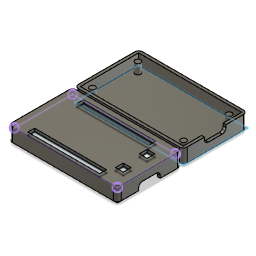
esp32-case (Autodesk Fusion 360 design; units mm, degrees)
Autodesk Fusion 360 part; units mm, degrees
sketch "Sketch1" plane through (0, 0, 0) normal (0, 1, 0) x (1, 0, 0)
  line L0 (-2, 31) -> (54, 31)
  line L1 (54, 31) -> (54, -2)
  line L2 (54, -2) -> (-2, -2)
  line L3 (-2, -2) -> (-2, 31)
  constraint horizontal L0
  constraint vertical L1
  constraint horizontal L2
  constraint vertical L3
extrude "Extrude1" add sketch "Sketch1" along normal blind 7 makes body 1
shell "Shell1" thickness 1.5 removed faces 1 at (16.6667, 7, -9) on bodies 1
cylinder "CylinderPrimitive1" add diameter 3.8 height 0.5 placed x (1, 0, 0) y (0, 0, -1) z (0, 1, 0) at (48.5, 1.5, -3.5) bodies 1
cylinder "CylinderPrimitive2" add diameter 3.8 height 3 placed x (1, 0, 0) y (0, 0, -1) z (0, 1, 0) at (48.5, 2, -3.5) bodies 1
cylinder "CylinderPrimitive3" add diameter 3 height 3 placed x (1, 0, 0) y (0, 0, -1) z (0, 1, 0) at (48.4953, 1.5, -25.4804) bodies 1
cylinder "CylinderPrimitive4" add diameter 4 height 3 placed x (1, 0, 0) y (0, 0, -1) z (0, 1, 0) at (3.5, 1.5, -25.5) bodies 1
cylinder "CylinderPrimitive5" add diameter 4 height 3 placed x (1, 0, 0) y (0, 0, -1) z (0, 1, 0) at (3.5, 1.5, -3.5) bodies 1
sketch "Sketch9" plane through (54, 0, 0) normal (1, 0, 0) x (0, 0, -1)
  line L0 (-2, 0) -> (31, 0)
  line L1 (31, 0) -> (31, 7)
  line L2 (31, 7) -> (-2, 7)
  line L3 (-2, 7) -> (-2, 0)
  line L4 (8.8903, 7) -> (8.8903, 3.7356)
  line L5 (8.8903, 3.7356) -> (20, 3.7356)
  line L6 (20, 3.7356) -> (20, 7)
  constraint coincident L2 L4.start
  constraint perpendicular L2 L4
  constraint perpendicular L4 L5
  constraint coincident L2 L6.end
  constraint perpendicular L2 L6
extrude "Extrude2" cut sketch "Sketch9" against normal blind 2 contours L2 L4 L5 L6 bodies 1
delete_face "DeleteFace1" 2 faces at (49.3668, 2.6667, -5.1908) (49.3708, 5, -2.73) on bodies 1
cylinder "CylinderPrimitive6" add diameter 4 height 3 placed x (1, 0, 0) y (0, 0, -1) z (0, 1, 0) at (48.5, 1.5, -3.5) bodies 1
delete_face "DeleteFace2" 2 faces at (48.9113, 4.5, -25.6035) (48.973, 3.5, -26.9023) on bodies 1
delete_face "DeleteFace3" 6 faces at (48.4118, 4.5, -3.9967) (50.4975, 2.5, -3.4003) (4.4276, 4.5, -2.8352) (5.4975, 2.5, -3.4003) (4.209, 4.5, -25.3143) (5.4901, 3.5, -25.3009) on bodies 1
cylinder "CylinderPrimitive7" add diameter 2.9 height 3 placed x (1, 0, 0) y (0, 0, -1) z (0, 1, 0) at (49.7786, 1.5, -2.3192) bodies 1
cylinder "CylinderPrimitive8" add diameter 2.9 height 3 placed x (1, 0, 0) y (0, 0, -1) z (0, 1, 0) at (2.2734, 1.5, -2.2495) bodies 1
cylinder "CylinderPrimitive9" add diameter 2.9 height 3 placed x (1, 0, 0) y (0, 0, -1) z (0, 1, 0) at (49.7438, 1.5, -26.8032) bodies 1
cylinder "CylinderPrimitive10" add diameter 2.9 height 3 placed x (1, 0, 0) y (0, 0, -1) z (0, 1, 0) at (2.2594, 1.5, -26.7528) bodies 1
delete_face "DeleteFace4" 4 faces at (49.9955, 2.5, -28.2312) (49.1847, 4.5, -27.2696) (50.0304, 2.5, -3.7472) (49.1826, 4.5, -2.7643) on bodies 1
delete_face "DeleteFace5" 4 faces at (3.7162, 3.5, -2.1052) (1.7425, 4.5, -2.8841) (3.7076, 2.5, -26.6805) (1.7285, 4.5, -27.3874) on bodies 1
cylinder "CylinderPrimitive11" add diameter 2.9 height 5 placed x (1, 0, 0) y (0, 0, -1) z (0, 1, 0) at (2.6, 1.5, -26) bodies 1
cylinder "CylinderPrimitive12" add diameter 2.9 height 5 placed x (1, 0, 0) y (0, 0, -1) z (0, 1, 0) at (2.6, 1.5, -2.6) bodies 1
cylinder "CylinderPrimitive13" add diameter 2.9 height 5 placed x (1, 0, 0) y (0, 0, -1) z (0, 1, 0) at (49.6109, 1.5, -2.5905) bodies 1
cylinder "CylinderPrimitive14" add diameter 2.9 height 5 placed x (1, 0, 0) y (0, 0, -1) z (0, 1, 0) at (49.6, 1.5, -26) bodies 1
fillet "Fillet1" radius 2 1 edges at (54, 3.5, -31) on bodies 1
fillet "Fillet2" radius 2 1 edges at (-2, 3.5, -31) on bodies 1
fillet "Fillet3" radius 2 1 edges at (-2, 3.5, 2) on bodies 1
fillet "Fillet4" radius 2 1 edges at (54, 3.5, 2) on bodies 1
fillet "Fillet5" radius 2 1 edges at (53.25, 3.7356, -8.8903) on bodies 1
fillet "Fillet6" radius 2 1 edges at (53.25, 3.7356, -20) on bodies 1
copy_body "CopyPasteBodies1" bodies 1 makes body 2
move_body "Move1" bodies 2 to x (1, 0, 0) y (0, -1, 0) z (0, 0, -1) at (0, 7, 5)
copy_body "Body->Comp1" bodies 2 removing the originals makes body 3 in component "Lid"
sketch "Sketch28" plane through (0, 5.5, 0) normal (0, -1, 0) x (1, 0, 0)
  circle A0 centre (49.6, 31) radius 1.45
  circle A1 centre (49.6109, 7.5905) radius 1.45
  circle A2 centre (2.6, 7.6) radius 1.45
  circle A3 centre (2.6, 31) radius 1.45
  line L0 (-0.5, 4.5) -> (52.5, 4.5)
  line L1 (52.5, 4.5) -> (52.5, 34.5)
  line L2 (52.5, 34.5) -> (-0.5, 34.5)
  line L3 (-0.5, 34.5) -> (-0.5, 4.5)
  line L4 (-0.5, 34.5) -> (2.6, 34.5)
  line L5 (2.6, 34.5) -> (2.6, 31)
  line L6 (2.6, 31) -> (-0.5, 31)
  line L7 (-0.5, 31) -> (-0.5, 34.5)
  circle A4 centre (2.6, 31) radius 1.45
  line L8 (2.6, 7.6) -> (-0.5, 7.6)
  line L9 (-0.5, 7.6) -> (-0.5, 4.5)
  line L10 (-0.5, 4.5) -> (2.6, 4.5)
  line L11 (2.6, 4.5) -> (2.6, 7.6)
  line L12 (49.6, 31) -> (52.5, 31)
  line L13 (52.5, 31) -> (52.5, 34.5)
  line L14 (52.5, 34.5) -> (49.6, 34.5)
  line L15 (49.6, 34.5) -> (49.6, 31)
  line L16 (49.6109, 7.5905) -> (52.5, 7.5905)
  line L17 (52.5, 7.5905) -> (52.5, 4.5)
  line L18 (52.5, 4.5) -> (49.6109, 4.5)
  line L19 (49.6109, 4.5) -> (49.6109, 7.5905)
  dimension "d47" = 3.1
  dimension "d48" = 3.5
  constraint horizontal L4
  constraint vertical L5
  constraint horizontal L6
  constraint vertical L7
  constraint coincident L2.end L3.start
  constraint concentric A3 A4
  constraint horizontal L8
  constraint vertical L9
  constraint horizontal L10
  constraint vertical L11
  constraint coincident L0.start L3.end
  constraint coincident A2.centre L8.start
  constraint horizontal L12
  constraint vertical L13
  constraint horizontal L14
  constraint vertical L15
  constraint coincident L1.end L2.start
  constraint coincident A0.centre L12.start
  constraint horizontal L16
  constraint vertical L17
  constraint horizontal L18
  constraint vertical L19
  constraint coincident L0.end L1.start
  constraint coincident A1.centre L16.start
  measures "d47" distance of L2.end L4.end
  measures "d48" distance of L2.end L6.end
extrude "Extrude2'" add sketch "Sketch28" along normal blind 7 contours A0 L1 L2 L12 L13 L14 L15 | A1 L0 L1 L16 L17 L18 L19 | A3 L2 L3 L4 L5 L6 L7 A4 | A2 L0 L3 L8 L9 L10 L11 bodies 3 in component "Lid"
delete_face "DeleteFace1'" 1 faces at (49.4688, 2.1667, 6.1475) on bodies 3 in component "Lid"
delete_face "DeleteFace2'" 1 faces at (51.043, 2.1667, 30.8579) on bodies 3 in component "Lid"
delete_face "DeleteFace3'" 1 faces at (4.05, 3.8333, 31) on bodies 3 in component "Lid"
delete_face "DeleteFace4'" 1 faces at (3.3454, 3.8333, 8.8437) on bodies 3 in component "Lid"
sketch "Sketch29" plane through (0, 5.5, 0) normal (0, -1, 0) x (1, 0, 0)
  line L0 (6.3, 34.4) -> (43.3, 34.4)
  line L1 (43.3, 34.4) -> (43.3, 30.9)
  line L2 (43.3, 30.9) -> (6.3, 30.9)
  line L3 (6.3, 30.9) -> (6.3, 34.4)
  line L4 (6.3, 9.1) -> (43.3, 9.1)
  line L5 (43.3, 9.1) -> (43.3, 5.6)
  line L6 (43.3, 5.6) -> (6.3, 5.6)
  line L7 (6.3, 5.6) -> (6.3, 9.1)
  line L8 (-0.5, 34.5) -> (-0.5, 4.5)
  line L9 (52.5, 34.5) -> (-0.5, 34.5)
  line L10 (-0.5, 4.5) -> (52.5, 4.5)
  line L11 (52.5, 4.5) -> (52.5, 34.5)
  line L12 (44.7, 27.63) -> (48.7, 27.63)
  line L13 (48.7, 27.63) -> (48.7, 23.63)
  line L14 (48.7, 23.63) -> (44.7, 23.63)
  line L15 (44.7, 23.63) -> (44.7, 27.63)
  line L16 (44.7, 15.37) -> (48.7, 15.37)
  line L17 (48.7, 15.37) -> (48.7, 11.37)
  line L18 (48.7, 11.37) -> (44.7, 11.37)
  line L19 (44.7, 11.37) -> (44.7, 15.37)
  dimension "d53" = 37
  dimension "d54" = 3.5
  dimension "d55" = 37
  dimension "d56" = 3.5
  dimension "d57" = 6.8
  dimension "d58" = 6.8
  dimension "d59" = 0.1
  dimension "d60" = 1.1
  dimension "d88" = 4
  dimension "d89" = 4
  dimension "d90" = 6.87
  dimension "d91" = 3.8
  dimension "d99" = 4
  dimension "d100" = 4
  dimension "d101" = 3.8
  dimension "d102" = 6.87
  constraint horizontal L0
  constraint vertical L1
  constraint horizontal L2
  constraint vertical L3
  constraint horizontal L4
  constraint vertical L5
  constraint horizontal L6
  constraint vertical L7
  constraint horizontal L12
  constraint vertical L13
  constraint horizontal L14
  constraint vertical L15
  constraint horizontal L16
  constraint vertical L17
  constraint horizontal L18
  constraint vertical L19
  measures "d53" distance of L0.start L0.end
  measures "d54" distance of L0.start L2.end
  measures "d55" distance of L4.start L4.end
  measures "d56" distance of L4.start L6.end
  measures "d57" distance of L3 L8
  measures "d58" distance of L7 L8
  measures "d59" distance of L0 L9
  measures "d60" distance of L6 L10
  measures "d88" distance of L12.start L12.end
  measures "d89" distance of L12.start L14.end
  measures "d90" distance of L9 L12
  measures "d91" distance of L11 L13
  measures "d99" distance of L16.start L16.end
  measures "d100" distance of L16.start L18.end
  measures "d101" distance of L11 L17
  measures "d102" distance of L10 L18
extrude "Extrude10" cut sketch "Sketch29" against normal blind 3 contours L0 L1 L2 L3 | L4 L5 L6 L7 | L12 L13 L14 L15 | L16 L17 L18 L19 bodies 3 in component "Lid"
extrude "Extrude9" cut sketch "Sketch29" against normal blind 3 contours L0 L1 L2 L3 | L4 L5 L6 L7 | L12 L13 L14 L15 bodies 3 in component "Lid"
component "Lid" placed x (1, 0, 0) y (0, 1, 0) z (0, 0, 1) at (0, 0, 0)
